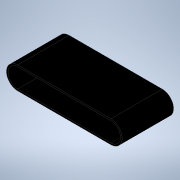
# Autodesk Inventor part: Shooting_Belt_2
Saved by Autodesk Inventor 2020 (Build 240168000, 168)
## iProperties
Created: 2022-01-27
Part Number: Shooting_Belt_2
Material: Generic
Document SubType Name: Modeling
Designer: danie
Density: 1 g/cm^3
Appearance: Default
Author: danie
Autodesk Inventor part; units mm, degrees
ref_plane "YZ Plane" through (0, 0, 0) normal (1, 0, 0) x (0, 1, 0)
ref_plane "XZ Plane" through (0, 0, 0) normal (0, 1, 0) x (-1, 0, 0)
ref_plane "XY Plane" through (0, 0, 0) normal (0, 0, 1) x (1, 0, 0)
sketch "Sketch1" plane through (0, 0, 0) normal (0, 0, 1) x (1, 0, 0)
  line L0 (0, 0) -> (-222.25, 0) construction
  line L1 (-19.05, 19.05) -> (-203.2, 19.05)
  line L2 (-203.2, -19.05) -> (-19.05, -19.05)
  arc A0 (-19.05, -19.05) -> (-19.05, 19.05) centre (-19.05, 0) ccw
  arc A1 (-203.2, 19.05) -> (-203.2, -19.05) centre (-203.2, 0) ccw
  line L3 (0, 0) -> (222.25, 0) construction
  line L4 (-203.2, 22.225) -> (-19.05, 22.225)
  arc A2 (-19.05, -22.225) -> (-19.05, 22.225) centre (-19.05, 0) ccw
  line L5 (-19.05, -22.225) -> (-203.2, -22.225)
  arc A3 (-203.2, 22.225) -> (-203.2, -22.225) centre (-203.2, 0) ccw
  point P0 (-111.125, 0)
  dimension "d0" = 222.25
  dimension "d1" = 180
  dimension "d2" = 38.1
  dimension "d3" = 3.175
  constraints: 14 end point, 10 point on circle, 4 centre point, 4 tangent, 2 horizontal, 2 parallel, 2 point on line, 1 collinear, 1 midpoint, 3 other
  measures "d0" distance of L0.start L0.end
  measures "d1" angle of L0 L3
  measures "d2" diameter of A1
  measures "d3" distance between parallel lines of L1 L4
extrude "Extrusion1" add sketch "Sketch1" along normal blind 101.6
body "Solid1"
